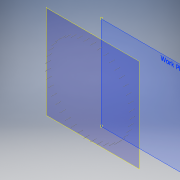
# Autodesk Inventor part: WheelConnectionPoleAJB
Saved by Autodesk Inventor 2018 (Build 220112000, 112)
## iProperties
Created: 2018-02-16
Part Number: WheelConnectionPoleAJB
Material: Generic
Document SubType Name: Modeling
Designer: Alec temporary
Density: 1 g/cm^3
Appearance: Default
Author: Alec temporary
Autodesk Inventor part; units mm, degrees
ref_plane "YZ Plane" through (0, 0, 0) normal (1, 0, 0) x (0, 1, 0)
ref_plane "XZ Plane" through (0, 0, 0) normal (0, 1, 0) x (-1, 0, 0)
ref_plane "XY Plane" through (0, 0, 0) normal (0, 0, 1) x (1, 0, 0)
ref_plane "Work Plane1" through (-16777.8073, 3410.1992, 12932.353) normal (0, 0, -1) x (-1, 0, 0)
sketch "Sketch1" plane through (-16777.8073, 3410.1992, 12932.353) normal (0, 0, -1) x (-1, 0, 0)
  spline S0 degree 3 poles (1787.5963, -22713.5651) (1796.933, -22712.8303) (1806.2285, -22713.8219) (1823.8007, -22718.9951) (1831.9195, -22723.0743) (1845.5285, -22733.2145) (1851.1813, -22739.0026) (1859.0635, -22750.172) (1861.7949, -22755.1133) (1865.1558, -22763.2184) (1866.1736, -22766.1708) (1867.7403, -22771.8258) (1868.3297, -22774.5064) (1869.0711, -22779.0348) (1869.3028, -22780.863) (1869.6271, -22784.4651) (1869.7243, -22786.2362) (1869.8079, -22790.4203) (1869.7415, -22792.8298) (1869.1606, -22800.574) (1868.1998, -22805.834) (1864.1201, -22819.7731) (1859.9747, -22828.0001) (1848.4945, -22843.301) (1840.9093, -22850.0977) (1824.1853, -22859.925) (1815.3515, -22863.1587) (1797.0673, -22866.1927) (1787.9629, -22866.0592) (1770.0263, -22862.5855) (1761.4423, -22859.2176) (1746.5837, -22850.0953) (1740.2189, -22844.5735) (1730.6222, -22832.9803) (1727.0373, -22827.2763) (1722.1773, -22816.6133) (1720.5572, -22811.8887) (1718.857, -22804.6778) (1718.416, -22802.3121) (1717.8457, -22798.171) (1717.6652, -22796.4072) (1717.4227, -22792.7982) (1717.366, -22790.955) (1717.3912, -22786.3595) (1717.5553, -22783.6142) (1718.6356, -22774.1527) (1720.2926, -22767.5981) (1726.1714, -22752.8148) (1731.0778, -22744.9933) (1743.9358, -22730.8587) (1752.0993, -22724.8087) (1769.518, -22716.6571) (1778.4076, -22714.2883) (1787.5963, -22713.5651) knots -48.628129 -48.628129 -48.628129 -48.628129 -45.818477 -45.818477 -43.059709 -43.059709 -40.592576 -40.592576 -38.879476 -38.879476 -37.937375 -37.937375 -37.112282 -37.112282 -36.559036 -36.559036 -36.026603 -36.026603 -35.302415 -35.302415 -33.690511 -33.690511 -30.897392 -30.897392 -27.805121 -27.805121 -24.973301 -24.973301 -22.23931 -22.23931 -19.448539 -19.448539 -16.87872 -16.87872 -14.832246 -14.832246 -13.326516 -13.326516 -12.60349 -12.60349 -12.071274 -12.071274 -11.517677 -11.517677 -10.690972 -10.690972 -8.650094 -8.650094 -5.844294 -5.844294 -2.765135 -2.765135 0 0 0 0 construction
  spline S1 degree 3 poles (1787.5963, -22720.8531) (1796.933, -22720.1183) (1806.2285, -22721.1098) (1823.8007, -22726.2831) (1831.9195, -22730.3622) (1845.5285, -22740.5024) (1851.1813, -22746.2905) (1859.0635, -22757.46) (1861.7949, -22762.4012) (1865.1558, -22770.5064) (1866.1736, -22773.4587) (1867.7403, -22779.1137) (1868.3297, -22781.7943) (1869.0711, -22786.3227) (1869.3028, -22788.1509) (1869.6271, -22791.7531) (1869.7243, -22793.5241) (1869.8079, -22797.7082) (1869.7415, -22800.1177) (1869.1606, -22807.8619) (1868.1998, -22813.122) (1864.1201, -22827.061) (1859.9747, -22835.288) (1848.4945, -22850.5889) (1840.9093, -22857.3857) (1824.1853, -22867.213) (1815.3515, -22870.4466) (1797.0673, -22873.4806) (1787.9629, -22873.3472) (1770.0263, -22869.8735) (1761.4423, -22866.5055) (1746.5837, -22857.3833) (1740.2189, -22851.8614) (1730.6222, -22840.2683) (1727.0373, -22834.5643) (1722.1773, -22823.9013) (1720.5572, -22819.1766) (1718.857, -22811.9657) (1718.416, -22809.6) (1717.8457, -22805.4589) (1717.6652, -22803.6951) (1717.4227, -22800.0861) (1717.366, -22798.2429) (1717.3912, -22793.6474) (1717.5553, -22790.9021) (1718.6356, -22781.4407) (1720.2926, -22774.886) (1726.1714, -22760.1027) (1731.0778, -22752.2812) (1743.9358, -22738.1467) (1752.0993, -22732.0966) (1769.518, -22723.945) (1778.4076, -22721.5762) (1787.5963, -22720.8531) knots -48.628129 -48.628129 -48.628129 -48.628129 -45.818477 -45.818477 -43.059709 -43.059709 -40.592576 -40.592576 -38.879476 -38.879476 -37.937375 -37.937375 -37.112282 -37.112282 -36.559036 -36.559036 -36.026603 -36.026603 -35.302415 -35.302415 -33.690511 -33.690511 -30.897392 -30.897392 -27.805121 -27.805121 -24.973301 -24.973301 -22.23931 -22.23931 -19.448539 -19.448539 -16.87872 -16.87872 -14.832246 -14.832246 -13.326516 -13.326516 -12.60349 -12.60349 -12.071274 -12.071274 -11.517677 -11.517677 -10.690972 -10.690972 -8.650094 -8.650094 -5.844294 -5.844294 -2.765135 -2.765135 0 0 0 0 construction
  circle A0 centre (1793.8618, -22793.1749) radius 79.8559
  line L0 (-32252.92, 0) -> (32252.92, 0) construction
  line L1 (0, -32252.92) -> (0, 32252.92) construction
  line L2 (0, 0) -> (1793.8618, -22793.1749) construction
  circle A1 centre (5337.4145, -22231.9313) radius 79.8559
  circle A2 centre (8749.5423, -21123.2637) radius 79.8559
  circle A3 centre (11946.2274, -19494.4713) radius 79.8559
  circle A4 centre (14848.7567, -17385.6603) radius 79.8559
  circle A5 centre (17385.6603, -14848.7567) radius 79.8559
  circle A6 centre (19494.4713, -11946.2274) radius 79.8559
  circle A7 centre (21123.2637, -8749.5423) radius 79.8559
  circle A8 centre (22231.9313, -5337.4145) radius 79.8559
  circle A9 centre (22793.1749, -1793.8618) radius 79.8559
  circle A10 centre (22793.1749, 1793.8618) radius 79.8559
  circle A11 centre (22231.9313, 5337.4145) radius 79.8559
  circle A12 centre (21123.2637, 8749.5423) radius 79.8559
  circle A13 centre (19494.4713, 11946.2274) radius 79.8559
  circle A14 centre (17385.6603, 14848.7567) radius 79.8559
  circle A15 centre (14848.7567, 17385.6603) radius 79.8559
  circle A16 centre (11946.2274, 19494.4713) radius 79.8559
  circle A17 centre (8749.5423, 21123.2637) radius 79.8559
  circle A18 centre (5337.4145, 22231.9313) radius 79.8559
  circle A19 centre (1793.8618, 22793.1749) radius 79.8559
  circle A20 centre (-1793.8618, 22793.1749) radius 79.8559
  circle A21 centre (-5337.4145, 22231.9313) radius 79.8559
  circle A22 centre (-8749.5423, 21123.2637) radius 79.8559
  circle A23 centre (-11946.2274, 19494.4713) radius 79.8559
  circle A24 centre (-14848.7567, 17385.6603) radius 79.8559
  circle A25 centre (-17385.6603, 14848.7567) radius 79.8559
  circle A26 centre (-19494.4713, 11946.2274) radius 79.8559
  circle A27 centre (-21123.2637, 8749.5423) radius 79.8559
  circle A28 centre (-22231.9313, 5337.4145) radius 79.8559
  circle A29 centre (-22793.1749, 1793.8618) radius 79.8559
  circle A30 centre (-22793.1749, -1793.8618) radius 79.8559
  circle A31 centre (-22231.9313, -5337.4145) radius 79.8559
  circle A32 centre (-21123.2637, -8749.5423) radius 79.8559
  circle A33 centre (-19494.4713, -11946.2274) radius 79.8559
  circle A34 centre (-17385.6603, -14848.7567) radius 79.8559
  circle A35 centre (-14848.7567, -17385.6603) radius 79.8559
  circle A36 centre (-11946.2274, -19494.4713) radius 79.8559
  circle A37 centre (-8749.5423, -21123.2637) radius 79.8559
  circle A38 centre (-5337.4145, -22231.9313) radius 79.8559
  circle A39 centre (-1793.8618, -22793.1749) radius 79.8559
  point P0 (-16777.8073, -3410.1992)
  point P1 (1787.5963, -22713.5651)
  point P2 (1787.5963, -22720.8531)
  dimension "d0" = 4.5
  dimension "d3" = 360
  constraints: 40 centre point, 6 end point, 1 horizontal, 1 midpoint, 1 vertical, 87 other
  measures "d0" angle of L1 L2
extrude "Extrusion1" add sketch "Sketch1" against normal blind 3048
body "Solid1"
